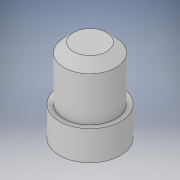
# Autodesk Inventor part: Knopf
Saved by Autodesk Inventor 2019 (Build 230136000, 136)
## iProperties
Created: 2020-06-14
Part Number: Knopf
Material: Generic
Document SubType Name: Modeling
Designer: Erle
Density: 1 g/cm^3
Appearance: Default
Author: Erle
Autodesk Inventor part; units mm, degrees
ref_plane "YZ Plane" through (0, 0, 0) normal (1, 0, 0) x (0, 1, 0)
ref_plane "XZ Plane" through (0, 0, 0) normal (0, 1, 0) x (-1, 0, 0)
ref_plane "XY Plane" through (0, 0, 0) normal (0, 0, 1) x (1, 0, 0)
sketch "Sketch1" plane through (0, 0, 0) normal (0, 1, 0) x (-1, 0, 0)
  circle A0 centre (0, 0) radius 2.8
  dimension "d0" = 5.6
  constraints: 1 centre point, 1 coincident
  measures "d0" diameter of A0
extrude "Extrusion1" add sketch "Sketch1" along normal blind 9
chamfer "Chamfer1" distance 1 angle 45 1 edges at (2.8, 9, 0)
sketch "Sketch3" plane through (0, 0, 0) normal (1, 0, 0) x (0, 1, 0)
  line L0 (0, -2.8) -> (8, -2.8) projected
  line L1 (3.2, -2.8) -> (0, -2.8)
  line L2 (0, -2.8) -> (0, -3.3)
  line L3 (0, -3.3) -> (3.2, -3.3)
  line L4 (3.2, -3.3) -> (3.2, -2.8)
  line L5 (0, 2.8) -> (0, -2.8) projected
  line L6 (-1.8, 0) -> (10.8, 0) projected
  point P0 (0, 0)
  dimension "d9" = 3.2
  dimension "d11" = 0.5
  constraints: 8 end point, 2 parallel, 1 horizontal, 1 perpendicular, 1 point on line, 1 vertical alignment
  measures "d9" distance between parallel lines of L5 L4
  measures "d11" distance of L3.end L1.start
revolve "Revolution1" add sketch "Sketch3" angle 360 about axis through (0, -10, 0) along (0, 1, 0)
body "Solid1"
